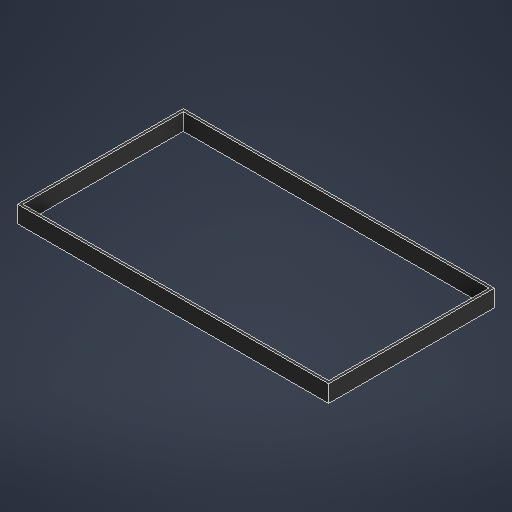
# Autodesk Inventor part: band
Saved by Autodesk Inventor 2025.2 (Build 292293000, 293)
## iProperties
Created: 2025-12-04
Part Number: band
Material: Rubber
Document SubType Name: Modeling
Designer: cloudy
Density: 0.93 g/cm^3
Appearance: Rubber - Black
Author: cloudy
Autodesk Inventor part; units mm, degrees
ref_plane "YZ Plane" through (0, 0, 0) normal (1, 0, 0) x (0, 1, 0)
ref_plane "XZ Plane" through (0, 0, 0) normal (0, 1, 0) x (-1, 0, 0)
ref_plane "XY Plane" through (0, 0, 0) normal (0, 0, 1) x (1, 0, 0)
sketch "Sketch1" plane through (0, 0, 0) normal (0, 1, 0) x (-1, 0, 0)
  line L0 (56.896, 29.845) -> (-56.896, 29.845)
  line L1 (-56.896, 29.845) -> (-56.896, -29.845)
  line L2 (-56.896, -29.845) -> (56.896, -29.845)
  line L3 (56.896, -29.845) -> (56.896, 29.845)
  line L4 (56.896, 29.845) -> (-56.896, -29.845) construction
  line L5 (-56.896, 29.845) -> (56.896, -29.845) construction
  line L6 (57.896, -30.845) -> (-57.896, -30.845)
  line L7 (-57.896, -30.845) -> (-57.896, 30.845)
  line L8 (-57.896, 30.845) -> (57.896, 30.845)
  line L9 (57.896, 30.845) -> (57.896, -30.845)
  point P0 (0, 0)
  dimension "d0" = 113.792
  dimension "d1" = 59.69
  dimension "d2" = 1
  constraints: 20 end point, 4 parallel, 2 midpoint, 2 perpendicular, 1 horizontal, 3 other
  measures "d0" distance of L2.end L1.end
  measures "d1" distance of L1.end L0.end
  measures "d2" distance between parallel lines of L2 L6
extrude "Extrusion1" add sketch "Sketch1" along normal blind 6.35
body "Solid1"
